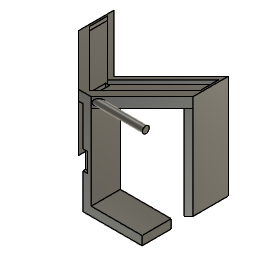
Mold upper corner left (Autodesk Fusion 360 design; units mm, degrees)
Autodesk Fusion 360 part; units mm, degrees
sketch "Sketch1" plane through (0, 0, 0) normal (0, 0, 1) x (1, 0, 0)
  line L0 (0, 0) -> (46.5, 0)
  line L1 (46.5, 0) -> (46.5, 23)
  line L2 (46.5, 23) -> (0, 23)
  line L3 (0, 23) -> (0, 0)
  dimension "d1" = 46.5
  dimension "d2" = 23
  constraint horizontal L0
  constraint vertical L1
  constraint horizontal L2
  constraint vertical L3
  constraint coincident L0.start L3.end
  measures "d1" distance of L0.start L0.end
  measures "d2" distance of L0.start L2.end
extrude "Extrude1" add sketch "Sketch1" along normal blind 7
sketch "Sketch2" plane through (0, 0, 7) normal (0, 0, 1) x (-1, 0, 0)
  line L0 (0, -23) -> (0, 0)
  line L1 (0, 0) -> (-46.5, 0)
  line L2 (-46.5, 0) -> (-46.5, -23)
  line L3 (-46.5, -23) -> (0, -23)
  line L4 (0, 0) -> (-6.5, 0)
  line L5 (-6.5, 0) -> (-6.5, -23)
  line L6 (-6.5, -23) -> (0, -23)
  line L7 (0, -23) -> (0, 0)
  dimension "d5" = 6.5
  dimension "d6" = 23
  constraint horizontal L4
  constraint vertical L5
  constraint horizontal L6
  constraint vertical L7
  constraint coincident L0.end L1.start
  measures "d5" distance of L0.end L4.end
  measures "d6" distance of L0.end L0.start
extrude "Extrude2" add sketch "Sketch2" along normal blind 67 contours L0 L1 L3 L4 L5 L6 L7
sketch "Sketch3" plane through (0, 0, 0) normal (-1, 0, 0) x (0, -1, 0)
  line L0 (-23, 0) -> (0, 0)
  line L1 (0, 0) -> (0, 74)
  line L2 (0, 74) -> (-23, 74)
  line L3 (-23, 74) -> (-23, 0)
  line L4 (-18, 74) -> (-5, 74)
  line L5 (-5, 74) -> (-5, 22)
  line L6 (-18, 74) -> (-18, 9)
  line L7 (-5, 22) -> (-18, 9)
  dimension "d9" = 13
  dimension "d10" = 52
  dimension "d11" = 65
  constraint perpendicular L3 L4
  constraint perpendicular L4 L5
  constraint vertical L6
  constraint coincident L2 L4.start
  measures "d9" distance of L4.start L4.end
  measures "d10" distance of L4.end L5.end
  measures "d11" distance of L4.start L6.end
extrude "Extrude3" cut sketch "Sketch3" against normal blind 3 contours L2 L4 L5 L6 L7
sketch "Sketch4" plane through (0, 0, 0) normal (-1, 0, 0) x (0, -1, 0)
  line L0 (-18, 9) -> (-18, 74)
  line L1 (-18, 74) -> (-23, 74)
  line L2 (-23, 74) -> (-23, 0)
  line L3 (-23, 0) -> (0, 0)
  line L4 (0, 0) -> (0, 74)
  line L5 (0, 74) -> (-5, 74)
  line L6 (-5, 74) -> (-5, 22)
  line L7 (-5, 22) -> (-18, 9)
  circle A0 centre (-20.268, 4) radius 1.75
  circle A1 centre (-2.732, 4) radius 1.75
  circle A2 centre (-20.268, 63) radius 1.75
  circle A3 centre (-2.732, 63) radius 1.75
  dimension "d14" = 3.5
  dimension "d15" = 3.5
  dimension "d16" = 3.5
  dimension "d17" = 3.5
  measures "d14" diameter of A0
  measures "d15" diameter of A1
  measures "d16" diameter of A2
  measures "d17" diameter of A3
extrude "Extrude4" cut sketch "Sketch4" against normal blind 3 contours A0 | A1 | A2 | A3
sketch "Sketch5" plane through (0, 0, 74) normal (0, 0, 1) x (-1, 0, 0)
  line L0 (0, -18) -> (-3, -18)
  line L1 (-3, -18) -> (-3, -5)
  line L2 (-3, -5) -> (0, -5)
  line L3 (0, -5) -> (0, 0)
  line L4 (0, 0) -> (-6.5, 0)
  line L5 (-6.5, 0) -> (-6.5, -23)
  line L6 (-6.5, -23) -> (0, -23)
  line L7 (0, -23) -> (0, -18)
  line L8 (-1.5, 5) -> (43.7548, -40.2548)
  line L9 (-1.5, -23) -> (43.7548, -68.2548)
  line L10 (43.7548, -40.2548) -> (43.7548, -68.2548)
  line L11 (-1.5, 5) -> (-46.7548, -40.2548)
  line L12 (-1.5, -23) -> (-46.7548, -68.2548)
  line L13 (-46.7548, -40.2548) -> (-46.7548, -68.2548)
  dimension "d21" = 64
  dimension "d22" = 64
  dimension "d25" = 64
  dimension "d27" = 64
  dimension "d28" = 90
  constraint coincident L6 L9.start
  constraint perpendicular L8 L11
  measures "d21" distance of L8.start L8.end
  measures "d22" distance of L9.start L9.end
  measures "d25" distance of L8.start L11.end
  measures "d27" distance of L9.start L12.end
  measures "d28" angle of L9 L12
sketch "Sketch6" plane through (0, 0, 74) normal (0, 0, 1) x (-1, 0, 0)
  line L0 (-1.5, -18, 8) -> (42.3406, -61.8406, 8)
  line L1 (-1.5, -3.5, 8) -> (42.3406, -47.3406, 8)
  line L2 (42.3406, -47.3406, 8) -> (42.3406, -61.8406, 8)
  line L3 (-1.5, -3.5, 8) -> (-45.3406, -47.3406, 8)
  line L4 (-1.5, -18, 8) -> (-45.3406, -61.8406, 8)
  line L5 (-45.3406, -47.3406, 8) -> (-45.3406, -61.8406, 8)
  dimension "d30" = 62
  dimension "d31" = 62
  dimension "d33" = 135
  dimension "d34" = 62
  dimension "d36" = 62
extrude "Extrude5" add sketch "Sketch5" along normal blind 8
extrude "Extrude6" cut sketch "Sketch6" against normal blind 3 contours L0 L1 L2 L3 L4 L5 in plane through (0, 0, 82) normal (0, 0, 1)
sketch "Sketch7" plane through (0, 0, 74) normal (0, 0, -1) x (1, 0, 0)
  line L0 (0, 0) -> (6.5, 0)
  line L1 (6.5, 0) -> (1.5, 5)
  line L2 (1.5, 5) -> (-43.7548, -40.2548)
  line L3 (-43.7548, -40.2548) -> (-43.7548, -68.2548)
  line L4 (-43.7548, -68.2548) -> (1.5, -23)
  line L5 (1.5, -23) -> (0, -23)
  line L6 (0, -23) -> (0, -18)
  line L7 (0, -18) -> (3, -18)
  line L8 (3, -18) -> (3, -5)
  line L9 (3, -5) -> (0, -5)
  line L10 (0, -5) -> (0, 0)
  line L11 (0, -5) -> (3, -5)
  line L12 (3, -5) -> (3, -18)
  line L13 (3, -18) -> (0, -18)
  line L14 (0, -18) -> (0, -5)
  constraint horizontal L11
  constraint vertical L12
  constraint horizontal L13
  constraint vertical L14
  constraint coincident L7.end L8.start
  constraint coincident L9.end L10.start
extrude "Extrude7" cut sketch "Sketch7" against normal blind 5 contours L7 L8 L9 L11 L12 L13 L14
sketch "Sketch8" plane through (0, 0, 74) normal (0, 0, -1) x (1, 0, 0)
  line L0 (6.5, 0) -> (6.5, -23)
  line L1 (6.5, -23) -> (1.5, -23)
  line L2 (1.5, -23) -> (46.7548, -68.2548)
  line L3 (46.7548, -68.2548) -> (46.7548, -40.2548)
  line L4 (46.7548, -40.2548) -> (6.5, 0)
  line L5 (46.7548, -68.2548) -> (43.2193, -64.7193)
  line L6 (43.2193, -64.7193) -> (43.2193, -36.7193)
  line L7 (43.2193, -36.7193) -> (46.7548, -40.2548)
  line L8 (46.7548, -40.2548) -> (46.7548, -68.2548)
  dimension "d43" = 5
  constraint coincident L2.end L3.start
  constraint coincident L2 L5.end
  constraint coincident L4 L6.end
  constraint vertical L6
  constraint coincident L3.end L4.start
  measures "d43" distance of L2.end L5.end
sketch "Sketch9" plane through (0, 0, 74) normal (0, 0, -1) x (1, 0, 0)
  line L0 (0, -18) -> (0, -5)
  line L1 (0, -5) -> (0, 0)
  line L2 (0, 0) -> (6.5, 0)
  line L3 (6.5, 0) -> (1.5, 5)
  line L4 (1.5, 5) -> (-43.7548, -40.2548)
  line L5 (-43.7548, -40.2548) -> (-43.7548, -68.2548)
  line L6 (-43.7548, -68.2548) -> (1.5, -23)
  line L7 (1.5, -23) -> (0, -23)
  line L8 (0, -23) -> (0, -18)
  line L9 (-43.7548, -68.2548) -> (-40.2193, -64.7193)
  line L10 (-40.2193, -64.7193) -> (-40.2193, -36.7193)
  line L11 (-40.2193, -36.7193) -> (-43.7548, -40.2548)
  line L12 (-43.7548, -40.2548) -> (-43.7548, -68.2548)
  dimension "d44" = 5
  constraint coincident L5.end L6.start
  constraint coincident L6 L9.end
  constraint coincident L4 L10.end
  constraint vertical L10
  constraint coincident L4.end L5.start
  measures "d44" distance of L5.end L9.end
extrude "Extrude8" add sketch "Sketch8" sketch "Sketch9" along normal blind 74 contours L2 L3 L4 L5 L6 L7 L8 of sketch 2 contours L4 L5 L6 L9 L10 L11 L12
sketch "Sketch10" plane through (0, 0, 74) normal (0, 0, -1) x (1, 0, 0)
  line L0 (-40.2193, -36.7193) -> (-40.2193, -64.7193)
  line L1 (-40.2193, -64.7193) -> (1.5, -23)
  line L2 (1.5, -23) -> (0, -23)
  line L3 (0, -23) -> (0, -18)
  line L4 (0, -18) -> (0, -5)
  line L5 (0, -5) -> (0, 0)
  line L6 (0, 0) -> (6.5, 0)
  line L7 (6.5, 0) -> (1.5, 5)
  line L8 (1.5, 5) -> (-40.2193, -36.7193)
  line L9 (6.5, 0) -> (-3.5, 0)
  line L10 (-3.5, 0) -> (1.5, 5)
  line L11 (1.5, 5) -> (6.5, 0)
  constraint coincident L6.end L7.start
  constraint coincident L8 L9.end
  constraint parallel L6 L9
  constraint coincident L7.end L8.start
extrude "Extrude9" cut sketch "Sketch10" against normal blind 8 contours L6 L7 L8 L9 L10 L11
move_face "OffsetFaces1" offset 0.255 1 faces at (46.5, 7.6667, 2.3333)
sketch "Sketch11" plane through (0, 0, 0) normal (1, 0, 0) x (0, 1, 0)
  circle A0 through (5.6925, 78, 6.5) (1.6538, 80.3318, 6.5) (1.6538, 75.6682, 6.5)
  dimension "d50" = 5.385
extrude "Extrude11" add sketch "Sketch11" along normal blind 40.255 contours A0 in plane through (6.5, 0, 0) normal (1, 0, 0)
sketch "Sketch12" plane through (0, 0, 0) normal (-1, 0, 0) x (0, -1, 0)
  circle A0 centre (-2.732, 63) radius 1.75
  circle A1 centre (-2.732, 4) radius 1.75
  circle A2 centre (-20.268, 63) radius 1.75
  circle A3 centre (-20.268, 4) radius 1.75
  line L0 (-18, 9) -> (-18, 74)
  line L1 (-18, 74) -> (-23, 74)
  line L2 (-23, 74) -> (-23, 0)
  line L3 (-23, 0) -> (0, 0)
  line L4 (0, 0) -> (0, 74)
  line L5 (0, 74) -> (-5, 74)
  line L6 (-5, 74) -> (-5, 22)
  line L7 (-5, 22) -> (-18, 9)
  line L8 (-21, 28) -> (-23, 28)
  line L9 (-23, 28) -> (-23, 43)
  line L10 (-23, 43) -> (-21, 43)
  line L11 (-21, 43) -> (-21, 28)
  line L12 (-2, 28) -> (0, 28)
  line L13 (0, 28) -> (0, 43)
  line L14 (0, 43) -> (-2, 43)
  line L15 (-2, 43) -> (-2, 28)
  dimension "d55" = 15
  dimension "d56" = 15
  constraint horizontal L8
  constraint vertical L9
  constraint horizontal L10
  constraint vertical L11
  constraint coincident L2 L9.end
  constraint horizontal L12
  constraint vertical L13
  constraint horizontal L14
  constraint vertical L15
  constraint coincident L4 L13.end
  measures "d55" distance of L8.start L10.end
  measures "d56" distance of L12.start L14.end
extrude "Extrude12" cut sketch "Sketch12" against normal blind 3.5 contours L2 L8 L9 L10 L11 | L4 L12 L13 L14 L15
